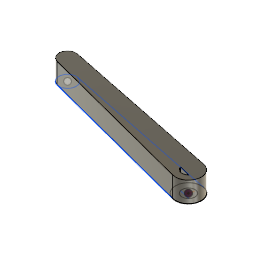
Hand-crank insert v3 (Autodesk Fusion 360 design; units mm, degrees)
Autodesk Fusion 360 part; units mm, degrees
note: some values were not read from the file. Set by a fixed rule: which sketch regions a step uses.
sketch "Sketch1" plane through (0, 0, 0) normal (0, 0, 1) x (1, 0, 0)
  circle A0 centre (0, 0) radius 10.75
  dimension "d1" = 21.5
  constraint coincident A0.centre origin
  measures "d1" diameter of A0
extrude "Extrude1" add sketch "Sketch1" along normal blind 114 makes body 1
sketch "Sketch2" plane through (0, 0, 114) normal (0, 0, 1) x (-1, 0, 0)
  circle A0 centre (0, 0) radius 10.75
  circle A1 centre (0, 0) radius 9.75
  dimension "d6" = 19.5
  constraint concentric A0 A1
  measures "d6" diameter of A1
extrude "Extrude2" cut sketch "Sketch2" against normal blind 2.5 contours A1 bodies 1
copy_body "CutPasteBodies1" bodies 1 removing the originals makes body 2 in component "Main Housing"
sketch "Sketch1 (2)" plane through (0, 0, 111.5) normal (0, 0, 1) x (-1, 0, 0) in component "Main Housing"
  circle A0 centre (0, 0) radius 9.75
  line L0 (-7.3121, -6.4494) -> (-7.3121, 6.4494)
  line L1 (7.3121, 6.4494) -> (7.3121, -6.4494)
  line L2 (7, -10.4909) -> (-7, 10.4909) construction
  line L3 (-7, -10.4909) -> (7, 10.4909) construction
  circle A1 centre (0, 0) radius 8.75
  circle A2 centre (7.25, 0) radius 2.5
  line L4 (7.3121, 0) -> (7.25, 0) construction
  line L5 (-0.1325, 8.749) -> (-0.1325, -8.749) construction
  circle A3 centre (-7.5149, 0) radius 2.5
  dimension "d9" = 14
  dimension "d14" = 5
  dimension "d15" = 17.5
  constraint parallel L0 L1
  constraint coincident L2 A0.centre
  constraint coincident L3 A0.centre
  constraint coincident A0.centre A1.centre
  constraint coincident A0 L1.end
  constraint coincident A0 L0.start
  constraint coincident A0 L0.end
  constraint coincident A0 L1.start
  constraint midpoint L1 L4.start
  constraint coincident A2.centre L4.end
  constraint perpendicular L1 L4
  constraint coincident A1 L5.start
  constraint coincident A1 L5.end
  constraint vertical L5
  constraint tangent A0 A2
  constraint symmetric A2 L5 A3
  measures "d9" distance of L2.end L3.end
  measures "d14" diameter of A2
  measures "d15" diameter of A1
extrude "Extrude1'" cut sketch "Sketch1 (2)" against normal up to surface (111.5 mm away) contours L1 A1 A2 | L1 A1 A2 | L1 A1 A2 | L1 A2 | L0 A1 A3 | L0 A1 A3 | L0 A1 A3 | L0 A3 bodies 2 in component "Main Housing"
extrude "Extrude4" cut sketch "Sketch1 (2)" against normal blind 9 contours L0 L1 A1 A2 A3 bodies 2 in component "Main Housing"
sketch "Sketch2 (2)" plane through (0, 0, 111.5) normal (0, 0, 1) x (-1, 0, 0) in component "Main Housing"
  line L0 (-4, -7.7822) -> (-4, 7.7822)
  line L1 (4, 7.7822) -> (4, -7.7822)
  line L2 (4, -12.291) -> (-4, 12.291) construction
  line L3 (-4, -12.291) -> (4, 12.291) construction
  circle A0 centre (0, 0) radius 8.75
  circle A1 centre (0, 0) radius 8.75
  line L4 (-4, -6.75) -> (4, -6.75)
  line L5 (4, -6.75) -> (4, 6.75)
  line L6 (4, 6.75) -> (-4, 6.75)
  line L7 (-4, 6.75) -> (-4, -6.75)
  line L8 (-4, -6.75) -> (4, 6.75) construction
  line L9 (4, -6.75) -> (-4, 6.75) construction
  dimension "d21" = 8
  dimension "d22" = 13.5
  constraint parallel L0 L1
  constraint coincident L2 A0.centre
  constraint coincident L3 A0.centre
  constraint coincident A0.centre A1.centre
  constraint perpendicular L4 L5
  constraint parallel L4 L6
  constraint parallel L5 L7
  constraint horizontal L4
  constraint coincident L8 A0.centre
  constraint coincident L9 A0.centre
  constraint coincident A0 L1.start
  constraint coincident A0 L0.end
  constraint coincident A0 L0.start
  constraint coincident A0 L1.end
  measures "d21" distance of L2.end L3.end
  measures "d22" distance of L4.end L5.end
extrude "Extrude5" add sketch "Sketch2 (2)" against normal up to surface (9 mm away) contours L0 L1 A0 A1 L4 | L0 L1 A0 A1 L6 bodies 2 in component "Main Housing"
sketch "Sketch1 (3)" plane through (0, 0, 114) normal (0, 0, 1) x (-1, 0, 0) in component "Cap"
  circle A0 centre (0, 0) radius 9.75
  circle A1 centre (0, 0) radius 10.75
  circle A2 centre (0, 0) radius 9.65
  circle A3 centre (0, 0) radius 3
  dimension "d25" = 19.3
  dimension "d28" = 6
  constraint coincident A0.centre A1.centre
  measures "d25" diameter of A2
  measures "d28" diameter of A3
extrude "Extrude1''" add sketch "Sketch1 (3)" against normal up to surface (2.5 mm away) separate body contours A2 makes body 3 in component "Cap"
sketch "Sketch1 (4)" plane through (0, 0, 0) normal (0, 0, 1) x (1, 0, 0) in component "Handle"
  circle A0 centre (0, 0) radius 6
  circle A1 centre (-73.0625, 16.9375) radius 4
  line L0 (-72.2634, 20.8568) -> (1.1986, 5.8791)
  line L1 (-74.0694, 13.0663) -> (-1.5104, -5.8068)
  circle A2 centre (0, 0) radius 3
  line L2 (-2.901, -0.7643) -> (2.1609, -2.081)
  line L3 (-0.37, -1.4227) -> (0.7552, 2.9034) construction
  dimension "d41" = 12
  dimension "d42" = 8
  dimension "d43" = 75
  dimension "d44" = 6
  dimension "d48" = 4.47
  constraint coincident A0.centre A2.centre
  constraint tangent A0 L0
  constraint tangent A1 L0
  constraint tangent A1 L1
  constraint tangent A0 L1
  constraint coincident A0 L0.end
  constraint coincident A0 L1.end
  constraint coincident A1 L1.start
  constraint coincident A1 L0.start
  constraint concentric A0 A2
  constraint coincident A2 L2.end
  constraint coincident A2 L2.start
  constraint parallel L1 L2
  constraint midpoint L2 L3.start
  constraint coincident A2 L3.end
  constraint perpendicular L2 L3
  measures "d41" diameter of A0
  measures "d42" diameter of A1
  measures "d43" distance of A0.centre A1.centre
  measures "d44" diameter of A2
  measures "d48" distance of L3.start L3.end
extrude "Extrude1'''" add sketch "Sketch1 (4)" along normal blind 2.5 separate body makes body 4 in component "Handle"
extrude "Extrude2'" add sketch "Sketch1 (4)" along normal blind 7 from surface at 2.5 contours A0 | A0 A1 L0 L1 | A1 | A2 L2 picked at (0.5427, 0.1152) bodies 4 in component "Handle"
component "Main Housing" placed x (1, 0, 0) y (0, 1, 0) z (0, 0, 1) at (0, 0, 0)
component "Cap" placed x (1, 0, 0) y (0, -1, 0) z (0, 0, -1) at (0, 0, 225.5)
component "Handle" placed x (1, 0, 0) y (0, 1, 0) z (0, 0, 1) at (0, 0, 0)
equation "d1 = diameter"
equation "d2 = length"
equation "diameter = 21.5 mm"
equation "length = 114 mm"
equation "d6 = diameter - 2 mm"
equation "d15 = diameter - 4 mm"
equation "d25 = diameter - 2.2 mm"
named bodies: "Test 1", "Main Body"
